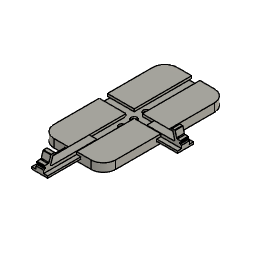
Modelo Dinamica De Estructuras Base Celular (Autodesk Fusion 360 design; units mm, degrees)
Autodesk Fusion 360 part; units mm, degrees
note: some values were not read from the file. Chosen so that the rebuilt part matches the saved one: which bodies a step acts on. Set by a fixed rule: which sketch regions a step uses.
sketch "Boceto1" plane through (0, 0, 0) normal (0, 0, 1) x (1, 0, 0)
  line L0 (37.5, 75) -> (-37.5, 75)
  line L1 (-37.5, 75) -> (-37.5, -75)
  line L2 (-37.5, -75) -> (37.5, -75)
  line L3 (37.5, -75) -> (37.5, 75)
  line L4 (37.5, 75) -> (-37.5, -75) construction
  line L5 (-37.5, 75) -> (37.5, -75) construction
  dimension "d1" = 75
  dimension "d2" = 150
  constraint horizontal L0
  constraint perpendicular L0 L1
  constraint parallel L0 L2
  constraint parallel L1 L3
  constraint coincident L4 origin
  constraint coincident L5 origin
  measures "d1" distance of L1.end L2.end
  measures "d2" distance of L0.end L1.end
extrude "Extruir1" add sketch "Boceto1" along normal blind 10 makes body 1
sketch "Boceto2" plane through (0, -75, 0) normal (0, -1, 0) x (1, 0, 0)
  line L0 (-37.5, 0) -> (37.5, 0)
  line L1 (37.5, 0) -> (37.5, 10)
  line L2 (37.5, 10) -> (-37.5, 10)
  line L3 (-37.5, 10) -> (-37.5, 0)
  line L4 (-5, 10) -> (5, 10)
  line L5 (5, 10) -> (5, 7)
  line L6 (5, 7) -> (-5, 7)
  line L7 (-5, 7) -> (-5, 10)
  line L8 (-10, 7) -> (10, 7)
  line L9 (10, 7) -> (10, 4)
  line L10 (10, 4) -> (-10, 4)
  line L11 (-10, 4) -> (-10, 7)
  line L12 (0, 7) -> (0, 10)
  line L13 (0, 4) -> (0, 7)
  dimension "d5" = 3
  dimension "d6" = 3
  dimension "d7" = 10
  dimension "d8" = 20
  constraint horizontal L4
  constraint vertical L5
  constraint horizontal L6
  constraint vertical L7
  constraint coincident L2 L4.start
  constraint horizontal L8
  constraint vertical L9
  constraint horizontal L10
  constraint vertical L11
  constraint midpoint L6 L12.start
  constraint midpoint L4 L12.end
  constraint midpoint L10 L13.start
  constraint midpoint L8 L12.start
  constraint midpoint L2 L12.end
  measures "d5" distance of L4.start L6.end
  measures "d6" distance of L8.start L10.end
  measures "d7" distance of L5.end L6.end
  measures "d8" distance of L8.start L8.end
extrude "Extruir2" cut sketch "Boceto2" against normal through all contours L2 L4 L6 L7 L8 L12 | L2 L4 L5 L6 L8 L12 | L6 L8 L10 L11 L13 | L6 L8 L9 L10 L13 bodies 1
sketch "Boceto3" plane through (37.5, 0, 0) normal (1, 0, 0) x (0, 1, 0)
  line L0 (-75, 0) -> (75, 0)
  line L1 (75, 0) -> (75, 10)
  line L2 (75, 10) -> (-75, 10)
  line L3 (-75, 10) -> (-75, 0)
  line L4 (-5, 10) -> (5, 10)
  line L5 (5, 10) -> (5, 7)
  line L6 (5, 7) -> (-5, 7)
  line L7 (-5, 7) -> (-5, 10)
  line L8 (-10, 7) -> (10, 7)
  line L9 (10, 7) -> (10, 4)
  line L10 (10, 4) -> (-10, 4)
  line L11 (-10, 4) -> (-10, 7)
  line L12 (0, 10) -> (0, 7)
  line L13 (0, 7) -> (0, 4)
  dimension "d11" = 3
  dimension "d12" = 3
  dimension "d13" = 10
  dimension "d14" = 20
  constraint horizontal L4
  constraint vertical L5
  constraint horizontal L6
  constraint vertical L7
  constraint coincident L2 L4.start
  constraint horizontal L8
  constraint vertical L9
  constraint horizontal L10
  constraint vertical L11
  constraint midpoint L4 L12.start
  constraint midpoint L6 L12.end
  constraint midpoint L8 L12.end
  constraint midpoint L10 L13.end
  constraint midpoint L2 L12.start
  measures "d11" distance of L4.start L6.end
  measures "d12" distance of L8.start L10.end
  measures "d13" distance of L5.end L6.end
  measures "d14" distance of L8.start L8.end
extrude "Extruir3" cut sketch "Boceto3" against normal through all contours L2 L4 L6 L7 L8 L12 | L2 L4 L5 L6 L8 L12 | L6 L8 L10 L11 L13 | L6 L8 L9 L10 L13 bodies 1
fillet "Empalme1" radius 15 4 edges at (37.5, -75, 5) (-37.5, -75, 5) (-37.5, 75, 5) (37.5, 75, 5) on bodies 1
sketch "Boceto4" plane through (0, 0, 4) normal (0, 0, 1) x (-1, 0, 0)
  line L0 (-10, -10) -> (-10, -75)
  line L1 (-10, -75) -> (10, -75)
  line L2 (10, -75) -> (10, -10)
  line L3 (10, -10) -> (37.5, -10)
  line L4 (37.5, -10) -> (37.5, 10)
  line L5 (37.5, 10) -> (10, 10)
  line L6 (10, 10) -> (10, 75)
  line L7 (10, 75) -> (-10, 75)
  line L8 (-10, 75) -> (-10, 10)
  line L9 (-10, 10) -> (-37.5, 10)
  line L10 (-37.5, 10) -> (-37.5, -10)
  line L11 (-37.5, -10) -> (-10, -10)
  circle A0 centre (0, 0) radius 2.25
  circle A1 centre (0, 15) radius 2.25
  circle A2 centre (0, -15) radius 2.25
  line L12 (0, 15) -> (0, -15)
  dimension "d19" = 4.5
  dimension "d20" = 15
  dimension "d21" = 15
  constraint coincident A0.centre origin
  constraint coincident A1.centre L12.start
  constraint coincident A2.centre L12.end
  constraint perpendicular L11 L12
  constraint coincident A0.centre L12
  constraint equal A0 A1
  constraint equal A0 A2
  measures "d19" diameter of A0
  measures "d20" vertical distance of A0.centre A1.centre
  measures "d21" vertical distance of A0.centre A2.centre
extrude "Extruir4" cut sketch "Boceto4" against normal through all contours A0 L12 | A0 L12 | A1 | A2 bodies 1
sketch "Boceto5" plane through (0, 0, 4) normal (0, 0, 1) x (-1, 0, 0)
  circle A0 centre (0, 15) radius 2.25
  circle A1 centre (0, 0) radius 2.25
  circle A2 centre (0, -15) radius 2.25
  line L0 (-10, -10) -> (-10, -75)
  line L1 (-10, -75) -> (10, -75)
  line L2 (10, -75) -> (10, -10)
  line L3 (10, -10) -> (37.5, -10)
  line L4 (37.5, -10) -> (37.5, 10)
  line L5 (37.5, 10) -> (10, 10)
  line L6 (10, 10) -> (10, 75)
  line L7 (10, 75) -> (-10, 75)
  line L8 (-10, 75) -> (-10, 10)
  line L9 (-10, 10) -> (-37.5, 10)
  line L10 (-37.5, 10) -> (-37.5, -10)
  line L11 (-37.5, -10) -> (-10, -10)
  circle A3 centre (0, 15) radius 4
  circle A4 centre (0, 0) radius 4
  circle A5 centre (0, -15) radius 4
  dimension "d23" = 8
  dimension "d24" = 8
  dimension "d25" = 8
  constraint concentric A0 A3
  constraint coincident A1.centre A4.centre
  constraint concentric A2 A5
  measures "d23" diameter of A3
  measures "d24" diameter of A4
  measures "d25" diameter of A5
extrude "Extruir5" cut sketch "Boceto5" against normal blind 2 contours A3 | A4 | A5 bodies 1
sketch "Boceto6" plane through (-37.5, 0, 0) normal (-1, 0, 0) x (0, -1, 0)
  line L0 (-60, 10) -> (-60, 0)
  line L1 (-60, 0) -> (60, 0)
  line L2 (60, 0) -> (60, 10)
  line L3 (60, 10) -> (5, 10)
  line L4 (5, 10) -> (5, 7)
  line L5 (5, 7) -> (10, 7)
  line L6 (10, 7) -> (10, 4)
  line L7 (10, 4) -> (-10, 4)
  line L8 (-10, 4) -> (-10, 7)
  line L9 (-10, 7) -> (-5, 7)
  line L10 (-5, 7) -> (-5, 10)
  line L11 (-5, 10) -> (-60, 10)
  line L12 (4.7, 6.7) -> (9.7, 6.7)
  line L13 (9.7, 6.7) -> (9.7, 4.3)
  line L14 (9.7, 4.3) -> (-9.7, 4.3)
  line L15 (-9.7, 4.3) -> (-9.7, 6.7)
  line L16 (-9.7, 6.7) -> (-4.7, 6.7)
  line L17 (-4.7, 6.7) -> (-4.7, 10.3)
  line L18 (-4.7, 10.3) -> (-60.3, 10.3)
  line L19 (-60.3, 10.3) -> (-60.3, -0.3)
  line L20 (-60.3, -0.3) -> (60.3, -0.3)
  line L21 (60.3, -0.3) -> (60.3, 10.3)
  line L22 (60.3, 10.3) -> (4.7, 10.3)
  line L23 (4.7, 10.3) -> (4.7, 6.7)
  line L24 (-4.7, 10.3) -> (4.7, 10.3)
  dimension "d28" = 0.3
extrude "Extruir6" add sketch "Boceto6" along normal blind -85 and the other way blind -10 separate body contours L12 L13 L14 L15 L16 L17 L23 L24 makes body 2
sketch "Boceto7" plane through (0, 75, 0) normal (0, 1, 0) x (-1, 0, 0)
  line L0 (-22.5, 10) -> (-22.5, 0)
  line L1 (-22.5, 0) -> (22.5, 0)
  line L2 (22.5, 0) -> (22.5, 10)
  line L3 (22.5, 10) -> (5, 10)
  line L4 (5, 10) -> (5, 7)
  line L5 (5, 7) -> (10, 7)
  line L6 (10, 7) -> (10, 4)
  line L7 (10, 4) -> (-10, 4)
  line L8 (-10, 4) -> (-10, 7)
  line L9 (-10, 7) -> (-5, 7)
  line L10 (-5, 7) -> (-5, 10)
  line L11 (-5, 10) -> (-22.5, 10)
  line L12 (-22.8, 10.3) -> (-22.8, -0.3)
  line L13 (-22.8, -0.3) -> (22.8, -0.3)
  line L14 (22.8, -0.3) -> (22.8, 10.3)
  line L15 (22.8, 10.3) -> (4.7, 10.3)
  line L16 (4.7, 10.3) -> (4.7, 6.7)
  line L17 (4.7, 6.7) -> (9.7, 6.7)
  line L18 (9.7, 6.7) -> (9.7, 4.3)
  line L19 (9.7, 4.3) -> (-9.7, 4.3)
  line L20 (-9.7, 4.3) -> (-9.7, 6.7)
  line L21 (-9.7, 6.7) -> (-4.7, 6.7)
  line L22 (-4.7, 6.7) -> (-4.7, 10.3)
  line L23 (-4.7, 10.3) -> (-22.8, 10.3)
  line L24 (-4.7, 10.3) -> (4.7, 10.3)
  dimension "d33" = 0.3
extrude "Extruir7" add sketch "Boceto7" along normal blind -160 and the other way blind -10 separate body contours L16 L17 L18 L19 L20 L21 L22 L24 makes body 3
sketch "Boceto8" plane through (0, 0, 0) normal (0, 0, 1) x (1, 0, 0)
  line L0 (-20, -20) -> (20, -20)
  line L1 (20, -20) -> (20, 20)
  line L2 (20, 20) -> (-20, 20)
  line L3 (-20, 20) -> (-20, -20)
  line L4 (-20, -20) -> (20, 20) construction
  line L5 (20, -20) -> (-20, 20) construction
  dimension "d38" = 40
  dimension "d39" = 40
  constraint horizontal L0
  constraint perpendicular L0 L1
  constraint parallel L0 L2
  constraint parallel L1 L3
  constraint coincident L4 origin
  constraint coincident L5 origin
  measures "d38" distance of L1.end L2.end
  measures "d39" distance of L0.end L1.end
extrude "Extruir8" cut sketch "Boceto8" along normal blind 40 bodies 2 3 makes body 5 at (-3.2333, -63.3333, 4.3) makes body 4 at (-29.1667, -3.2333, 4.3)
sketch "Boceto9" plane through (4.7, 0, 0) normal (1, 0, 0) x (0, 1, 0)
  line L0 (-20, 6.7) -> (-20, 10.3)
  line L1 (-20, 10.3) -> (-85, 10.3)
  line L2 (-85, 10.3) -> (-85, 6.7)
  line L3 (-85, 6.7) -> (-20, 6.7)
  line L4 (-85, 10.3) -> (-80, 10.3)
  line L5 (-76.8377, 10.3) -> (-73.5044, 20.3)
  line L6 (-73.5044, 20.3) -> (-71, 20.3)
  line L7 (-71, 20.3) -> (-71, 22.3)
  line L8 (-71, 22.3) -> (-76, 22.3)
  line L9 (-76, 22.3) -> (-80, 10.3)
  line L10 (-85, 10.3) -> (-82.5, 10.3)
  line L11 (-82.5, 12.3) -> (-84, 12.3)
  line L12 (-84, 12.3) -> (-84, 14.3)
  line L13 (-84, 14.3) -> (-78.6667, 14.3)
  line L14 (-82.5, 12.3) -> (-82.5, 10.3)
  dimension "d42" = 5
  dimension "d45" = 12
  dimension "d46" = 4
  dimension "d47" = 3
  dimension "d48" = 2
  dimension "d49" = 5
  dimension "d56" = 2
  dimension "d57" = 1.5
  dimension "d58" = 2
  constraint coincident L1.end L2.start
  constraint perpendicular L2 L4
  constraint coincident L1 L5.start
  constraint parallel L1 L6
  constraint perpendicular L1 L7
  constraint perpendicular L7 L8
  constraint parallel L5 L9
  constraint midpoint L4 L10.end
  constraint perpendicular L2 L11
  constraint perpendicular L11 L12
  constraint coincident L9 L13.end
  constraint perpendicular L12 L13
  constraint perpendicular L4 L14
  measures "d42" distance of L1.end L4.end
  measures "d45" vertical distance of L4.end L8.end
  measures "d46" horizontal distance of L4.end L8.end
  measures "d47" distance of L5 L9
  measures "d48" distance of L6 L8
  measures "d49" distance of L7.end L8.end
  measures "d56" distance of L11.end L12.end
  measures "d57" distance of L11.start L11.end
  measures "d58" distance of L10.end L11.start
extrude "Extruir9" add sketch "Boceto9" against normal up to surface (9.4 mm away) contours L1 L5 L6 L7 L8 L9 | L1 L4 L9 L11 L12 L13 L14 bodies 5
fillet "Empalme2" radius 1 2 edges at (0, -76.8377, 10.3) (0, -78.6667, 14.3) on bodies 5
fillet "Empalme3" radius 0.5 8 edges at (0, -71, 22.3) (0, -71, 20.3) (0, -73.5044, 20.3) (0, -76, 22.3) (0, -84, 12.3) (0, -84, 14.3) (0, -82.5, 12.3) (0, -82.5, 10.3) on bodies 5
sketch "Boceto10" plane through (0, 4.7, 0) normal (0, 1, 0) x (-1, 0, 0)
  line L0 (-20, 6.7) -> (-20, 10.3)
  line L1 (-20, 10.3) -> (-47.5, 10.3)
  line L2 (-47.5, 10.3) -> (-47.5, 6.7)
  line L3 (-47.5, 6.7) -> (-20, 6.7)
  line L4 (-42.5, 10.3) -> (-39.5, 22.3)
  line L5 (-39.5, 22.3) -> (-35.5, 22.3)
  line L6 (-35.5, 22.3) -> (-35.5, 20.3)
  line L7 (-35.5, 20.3) -> (-36.9077, 20.3)
  line L8 (-36.9077, 20.3) -> (-39.4077, 10.3)
  line L9 (-41.5, 14.3) -> (-46.5, 14.3)
  line L10 (-46.5, 14.3) -> (-46.5, 12.3)
  line L11 (-46.5, 12.3) -> (-45, 12.3)
  line L12 (-45, 12.3) -> (-45, 10.3)
  dimension "d59" = 2.5
  dimension "d60" = 5
  dimension "d61" = 3
  dimension "d62" = 12
  dimension "d63" = 2
  dimension "d64" = 3
  dimension "d65" = 4
  dimension "d66" = 2
  dimension "d67" = 1.5
  dimension "d68" = 2
  constraint coincident L1 L4.start
  constraint parallel L1 L5
  constraint perpendicular L5 L6
  constraint coincident L1 L8.end
  constraint coincident L4 L9.start
  constraint parallel L1 L9
  constraint perpendicular L9 L10
  constraint perpendicular L10 L11
  constraint coincident L1 L12.end
  constraint perpendicular L11 L12
  constraint parallel L4 L8
  constraint perpendicular L6 L7
  measures "d59" distance of L2 L12
  measures "d60" distance of L1.end L4.start
  measures "d61" horizontal distance of L4.start L4.end
  measures "d62" vertical distance of L4.start L4.end
  measures "d63" distance of L5.end L6.end
  measures "d64" distance of L4 L8
  measures "d65" distance of L4.end L5.end
  measures "d66" distance of L9.end L10.end
  measures "d67" distance of L10.end L11.end
  measures "d68" distance of L11.end L12.end
extrude "Extruir10" add sketch "Boceto10" against normal up to surface (9.4 mm away) contours L1 L4 L5 L6 L7 L8 | L1 L4 L9 L10 L11 L12 bodies 2
fillet "Empalme4" radius 1 2 edges at (39.4077, 0, 10.3) (41.5, 0, 14.3) on bodies 2
fillet "Empalme5" radius 0.5 7 edges at (35.5, 0, 20.3) (35.5, 0, 22.3) (39.5, 0, 22.3) (46.5, 0, 14.3) (46.5, 0, 12.3) (45, 0, 12.3) (45, 0, 10.3) on bodies 2
extrude "Extruir11" add 1 faces at (20, -1.5667, 7.9) along direction (-1, 0, 0) blind 15 on bodies 2 bodies 2
move_body "Desplazar1" bodies 2 to x (1, 0, 0) y (0, 1, 0) z (0, 0, 1) at (15, 0, 0)
move_body "Desplazar2" bodies 5 to x (1, 0, 0) y (0, 1, 0) z (0, 0, 1) at (0, -30, 0)
fillet "Empalme6" radius 3 4 edges at (20, -9.7, 5.5) (20, 9.7, 5.5) (-9.7, -50, 5.5) (9.7, -50, 5.5) on bodies 2 5
hidden bodies 3 4
named bodies: "Base Celular", "Lateral", "Frontal"
